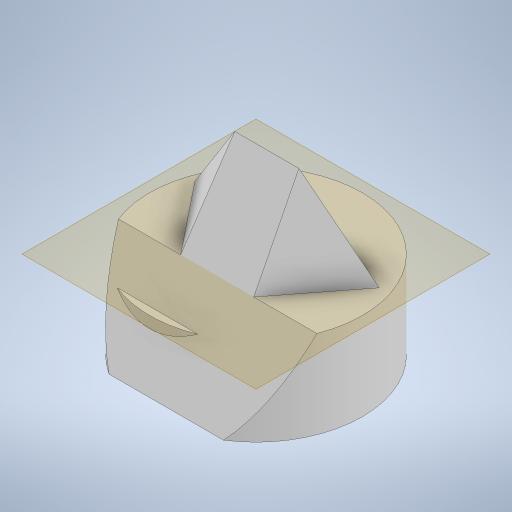
# Autodesk Inventor part: Даник
Saved by Autodesk Inventor 2024 (Build 280153000, 153)
## iProperties
Created: 2023-11-25
Part Number: Даник
Material: Типовые
Document SubType Name: Modeling
Designer: User
Density: 1 g/cm^3
Appearance: По умолчанию
Author: User
Autodesk Inventor part; units mm, degrees
ref_plane "YZ Plane" through (0, 0, 0) normal (1, 0, 0) x (0, 1, 0)
ref_plane "XZ Plane" through (0, 0, 0) normal (0, 1, 0) x (-1, 0, 0)
ref_plane "XY Plane" through (0, 0, 0) normal (0, 0, 1) x (1, 0, 0)
sketch "Эскиз1" plane through (0, 0, 0) normal (0, 1, 0) x (-1, 0, 0)
  circle A0 centre (0, 0) radius 30.3329
  constraints: 1 centre point, 1 coincident
extrude "Выдавливание1" add sketch "Эскиз1" along normal blind 25
sketch "Эскиз2" plane through (0, 25, 0) normal (0, 1, 0) x (1, 0, 0)
  line L0 (0, -24.1972) -> (-26.6685, 9.2514)
  line L1 (-26.6685, 9.2514) -> (25.8868, 9.2514)
  line L2 (25.8868, 9.2514) -> (0, -24.1972)
  point P0 (0, 0)
  point P1 (0, 0)
  constraints: 6 end point, 1 horizontal
ref_plane "РабПлоскость1" through (0, 25, 0) normal (0, 1, 0) x (1, 0, 0)
sketch "Эскиз6" plane through (0, 0, 0) normal (1, 0, 0) x (0, 1, 0)
  point P0 (0, 0)
  point P1 (61.9153, 0)
loft "Лофт3" add profiles "Эскиз2" section 1 point at (0, 61.9153, 0)
sketch "Эскиз7" plane through (0, 0, 0) normal (1, 0, 0) x (0, 1, 0)
  line L0 (61.9153, 0) -> (25, -9.2514) projected
  line L1 (49.0637, -3.2208) -> (0, 25.588)
  line L2 (0, -30.3329) -> (0, 30.3329) projected
  line L3 (0, 45.3133) -> (65.7508, 0)
  line L4 (65.7508, 0) -> (51.8075, -4.8318)
  line L5 (51.8075, -4.8318) -> (49.0637, -3.2208)
  line L6 (0, 45.3133) -> (0, 25.588)
  point P0 (0, 0)
  constraints: 10 end point, 3 point on line, 2 collinear
extrude "Выдавливание3" cut sketch "Эскиз7" along normal mid plane 356
